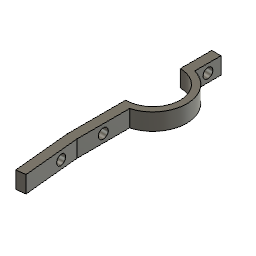
Trumpet+Clamp+2+Secondary (Autodesk Fusion 360 design; units mm, degrees)
Autodesk Fusion 360 part; units mm, degrees
sketch "Sketch1" plane through (0, 0, 0) normal (0, 1, 0) x (1, 0, 0)
  circle A0 centre (0, 0) radius 12.435
  circle A1 centre (0, 0) radius 15.435
  line L0 (0, 0) -> (-15.435, 0) construction
  line L1 (0, 0) -> (15.435, 0) construction
  line L2 (-4.25, -39.2475) -> (0.7697, -91.2632)
  line L3 (4.25, -38.8384) -> (9.2303, -90.4468)
  circle A2 centre (5, -90.855) radius 4.25
  line L4 (5, -90.855) -> (0.7697, -91.2632) construction
  line L5 (5, -90.855) -> (9.2303, -90.4468) construction
  circle A3 centre (5, -90.855) radius 2.25
  line L6 (-4.25, -39.2475) -> (-4.25, -14.8384)
  line L7 (4.25, -38.8384) -> (4.25, -14.8384)
  line L8 (0, 0) -> (0, -38.8384) construction
  line L9 (4.25, -38.8384) -> (-4.25, -38.8384) construction
  line L10 (-4.25, 14.8384) -> (-4.25, 26.8384)
  line L11 (-4.25, 26.8384) -> (4.25, 26.8384)
  line L12 (4.25, 26.8384) -> (4.25, 14.8384)
  line L13 (-4.25, -14.8384) -> (-4.25, 14.8384) construction
  line L14 (4.25, 14.8384) -> (4.25, -14.8384) construction
  line L15 (5, -90.855) -> (5, -95.105) construction
  point P0 (0, -15.435)
  point P1 (5, -95.105)
  dimension "d1" = 24.87
  dimension "d3" = 4.5
  dimension "d4" = 8.5
  dimension "d5" = 5
  dimension "d19" = 8.5
  dimension "d22" = 30.87
  dimension "d31" = 12
  dimension "d32" = 24
  dimension "d35" = 79.67
  constraint coincident A0.centre A1.centre
  constraint concentric A0 A1
  constraint coincident A1 L0.end
  constraint horizontal L0
  constraint coincident A1 L1.end
  constraint parallel L0 L1
  constraint coincident A2.centre L4.start
  constraint coincident A2 L2.end
  constraint coincident A2 L3.end
  constraint parallel L4 L5
  constraint coincident L2.end L4.end
  constraint coincident L3.end L5.end
  constraint coincident A1 L6.end
  constraint coincident A1 L7.end
  constraint parallel L2 L3
  constraint vertical L6
  constraint vertical L7
  constraint vertical L8
  constraint tangent L3 A2
  constraint coincident L6 L9.end
  constraint perpendicular L6 L9
  constraint midpoint L8.end L9
  constraint coincident A1 L10.start
  constraint vertical L10
  constraint perpendicular L10 L11
  constraint coincident A1 L12.end
  constraint perpendicular L11 L12
  constraint vertical L13
  constraint vertical L14
  constraint coincident L8 P0
  constraint coincident A1 P0
  constraint coincident A2 P1
  constraint vertical L15
  constraint coincident P1 L15.end
  measures "d1" diameter of A0
  measures "d3" diameter of A3
  measures "d4" diameter of A2
  measures "d5" horizontal distance of A0.centre A2.centre
  measures "d19" distance of L6 L7
  measures "d22" diameter of A1
  measures "d31" distance of L11.end L12.end
  measures "d32" distance of L3.start L7.end
  measures "d35" vertical distance of P0 P1
extrude "Extrude1" add sketch "Sketch1" along normal blind 7.7
sketch "Sketch2" plane through (0.4974, 0, -0.048) normal (0.995376, 0, -0.096056) x (-0.096056, 0, -0.995376)
  line L0 (-90.9152, 0) -> (-39.067, 0)
  line L1 (-39.067, 0) -> (-39.067, 7.7)
  line L2 (-39.067, 7.7) -> (-90.9152, 7.7)
  line L3 (-90.9152, 7.7) -> (-90.9152, 0)
  line L4 (-39.067, 3.85) -> (-90.9152, 3.85) construction
  circle A0 centre (-47.067, 3.85) radius 2.25
  dimension "d33" = 8
  dimension "d34" = 4.5
  constraint midpoint L1 L4.start
  constraint midpoint L3 L4.end
  constraint coincident L4 A0.centre
  measures "d33" distance of L1 A0.centre
  measures "d34" diameter of A0
extrude "Extrude2" cut sketch "Sketch2" against normal up to surface (8.5 mm away) contours A0
sketch "Sketch3" plane through (4.25, 0, 0) normal (1, 0, 0) x (0, 0, -1)
  line L0 (-38.8384, 0) -> (-14.8384, 0)
  line L1 (-14.8384, 0) -> (-14.8384, 7.7)
  line L2 (-14.8384, 7.7) -> (-38.8384, 7.7)
  line L3 (-38.8384, 7.7) -> (-38.8384, 0)
  line L4 (-14.8384, 3.85) -> (-38.8384, 3.85) construction
  circle A0 centre (-26.8384, 3.85) radius 2.25
  line L5 (14.8384, 0) -> (26.8384, 0) construction
  line L6 (26.8384, 0) -> (26.8384, 7.7) construction
  line L7 (26.8384, 7.7) -> (14.8384, 7.7) construction
  line L8 (14.8384, 7.7) -> (14.8384, 0) construction
  line L9 (14.8384, 3.85) -> (26.8384, 3.85) construction
  circle A1 centre (20.8384, 3.85) radius 2.25
  dimension "d16" = 4.5
  constraint midpoint L1 L4.start
  constraint midpoint L3 L4.end
  constraint midpoint L4 A0.centre
  constraint midpoint L8 L9.start
  constraint midpoint L6 L9.end
  constraint midpoint L9 A1.centre
  constraint equal A0 A1
  measures "d16" diameter of A0
extrude "Extrude3" cut sketch "Sketch3" against normal up to surface (8.5 mm away) contours A0 | A1
sketch "Sketch4" plane through (0, 0, 0) normal (1, 0, 0) x (0, 0, -1)
  circle A0 centre (-26.8384, 3.85) radius 2.25 construction
  line L0 (-38.8384, 0) -> (-14.8384, 0) construction
  line L1 (-14.8384, 0) -> (-14.8384, 7.7) construction
  line L2 (-14.8384, 7.7) -> (-38.8384, 7.7) construction
  line L3 (-38.8384, 7.7) -> (-38.8384, 0) construction
  line L4 (14.8384, 0) -> (-14.8384, 0) construction
  line L5 (-14.8384, 0) -> (-14.8384, 7.7) construction
  line L6 (14.8384, 7.7) -> (-14.8384, 7.7) construction
  line L7 (-14.8384, 7.7) -> (-14.8384, 0) construction
  circle A1 centre (-26.8384, 3.85) radius 2.25 construction
  line L8 (-14.8384, 0) -> (-39.2475, 0) construction
  line L9 (-39.2475, 0) -> (-39.2475, 7.7) construction
  line L10 (-39.2475, 7.7) -> (-14.8384, 7.7) construction
  line L11 (-14.8384, 7.7) -> (-14.8384, 0) construction
  line L12 (14.8384, 0) -> (-39.0429, 0)
  line L13 (-39.0429, 0) -> (-39.0429, 7.7)
  line L14 (-39.0429, 7.7) -> (14.8384, 7.7)
  line L15 (14.8384, 7.7) -> (14.8384, 0)
  line L16 (-39.2475, 7.7) -> (-38.8384, 7.7) construction
  line L17 (14.8384, 7.7) -> (14.8384, 0)
  line L18 (14.8384, 0) -> (-14.8384, 0)
  line L19 (14.8384, 0) -> (14.8384, 7.7)
  line L20 (14.8384, 7.7) -> (-14.8384, 7.7)
  circle A2 centre (20.8384, 3.85) radius 2.25
  line L21 (14.8384, 0) -> (26.8384, 0)
  line L22 (26.8384, 0) -> (26.8384, 7.7)
  line L23 (26.8384, 7.7) -> (14.8384, 7.7)
  line L24 (14.8384, 7.7) -> (14.8384, 0)
  constraint horizontal L12
  constraint vertical L13
  constraint horizontal L14
  constraint vertical L15
  constraint coincident L10 L13.end
  constraint coincident L4.start L12.start
  constraint coincident L9.end L10.start
  constraint coincident L2.end L3.start
  constraint midpoint L13.end L16
extrude "Extrude4" cut sketch "Sketch4" against normal blind 15.435
ref_plane "WorkPlane1" through (2.4902, 3.85, 64.8471) normal (-0.995376, 0, 0.096056) x (0.096056, 0, 0.995376)
sketch "Sketch5" plane through (-3.733, 0, 0.3602) normal (-0.995376, 0, 0.096056) x (0.096056, 0, 0.995376)
  line L0 (12.3775, 7.7) -> (12.3775, 0) construction
  line L1 (12.3775, 0) -> (38.8624, 0) construction
  line L2 (38.8624, 0) -> (38.8624, 7.7) construction
  line L3 (38.8624, 7.7) -> (12.3775, 7.7) construction
  ellipse E0 centre (26.7142, 3.85) end of major axis (26.7142, 1.6) minor radius 2.2396
  line L4 (88.6652, 7.7) -> (93.1652, 7.7) construction
  line L5 (38.8624, 7.7) -> (90.9152, 7.7) construction
  line L6 (90.9152, 7.7) -> (90.9152, 0) construction
  line L7 (90.9152, 0) -> (38.8624, 0) construction
  line L8 (38.8624, 0) -> (38.8624, 7.7) construction
  line L9 (64.8888, 7.7) -> (33.5308, 7.7)
  line L10 (33.5308, 7.7) -> (33.5308, 0)
  line L11 (33.5308, 0) -> (64.8888, 0)
  line L12 (64.8888, 0) -> (64.8888, 7.7)
  constraint horizontal L5
  constraint vertical L6
  constraint horizontal L7
  constraint vertical L8
  constraint coincident L2.end L3.start
  constraint midpoint L4 L5.end
  constraint coincident L1.end L7
  constraint horizontal L9
  constraint vertical L10
  constraint horizontal L11
  constraint vertical L12
  constraint coincident L1 L10.end
  constraint midpoint L5 L9.start
extrude "Extrude5" cut sketch "Sketch5" along normal up to surface (4.25 mm away) contours L9 L10 L11 L12
sketch "Sketch6" plane through (-7.9633, 0, 0.7685) normal (-0.995376, 0, 0.096056) x (0.096056, 0, 0.995376)
  line L0 (38.8624, 7.7) -> (38.8624, 0)
  line L1 (38.8624, 0) -> (64.8888, 0)
  line L2 (64.8888, 7.7) -> (38.8624, 7.7)
  circle A0 centre (47.067, 3.85) radius 2.25
  line L3 (64.8888, 7.7) -> (111.7152, 7.7)
  line L4 (111.7152, 7.7) -> (111.7152, 0)
  line L5 (111.7152, 0) -> (64.8888, 0)
  line L6 (64.8888, 0) -> (64.8888, 7.7)
  line L7 (64.8888, 0) -> (64.8888, 7.7)
  constraint horizontal L3
  constraint vertical L4
  constraint horizontal L5
  constraint vertical L6
  constraint coincident L2.start L3.start
  constraint coincident L1.end L5
extrude "Extrude6" cut sketch "Sketch6" against normal up to surface (8.5 mm away) contours L3 L4 L5 L6 L7
equation "d19 = d4"
equation "d20 = ( -d22 / 2 mm ) * 1 mm"
equation "d22 = d1 + 6 mm"
